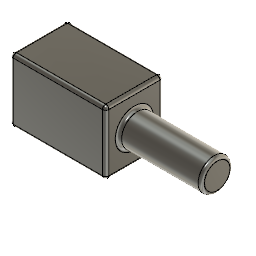
_Sign Holder (YIELD).780cf146-7897-4be0-9e8e-9a865215b20b (Autodesk Fusion 360 design; units mm, degrees)
Autodesk Fusion 360 part; units mm, degrees
sketch "Sketch1" plane through (0, 0, 0) normal (0, 0, 1) x (1, 0, 0)
  line L0 (0, 0) -> (-38.1, 0)
  line L1 (-38.1, 0) -> (-38.1, -38.1)
  line L2 (-38.1, -38.1) -> (0, -38.1)
  line L3 (0, -38.1) -> (0, 0)
  dimension "d1" = 38.1
  dimension "d2" = 38.1
  constraint horizontal L0
  constraint vertical L1
  constraint horizontal L2
  constraint vertical L3
  constraint coincident L0.start L3.end
  measures "d1" distance of L0.start L0.end
  measures "d2" distance of L0.start L2.end
extrude "Extrude1" add sketch "Sketch1" along normal blind 25.4
sketch "Sketch2" plane through (0, 0, 0) normal (1, 0, 0) x (0, 1, 0)
  line L0 (-38.1, 0) -> (0, 0)
  line L1 (0, 0) -> (0, 25.4)
  line L2 (0, 25.4) -> (-38.1, 25.4)
  line L3 (-38.1, 25.4) -> (-38.1, 0)
  line L4 (-38.1, 0) -> (-19.05, 0)
  line L5 (-19.05, 0) -> (-19.05, 12.7)
  circle A0 centre (-19.05, 12.7) radius 6.35
  dimension "d5" = 12.7
  constraint coincident L0.start L3.end
  constraint midpoint L0 L4.end
  constraint perpendicular L4 L5
  constraint coincident L5.end A0.centre
  measures "d5" diameter of A0
extrude "Extrude2" add sketch "Sketch2" along normal blind 12.7 contours A0
sketch "Sketch3" plane through (0, 0, 0) normal (0, 0, -1) x (1, 0, 0)
  line L0 (0, 0) -> (0, 38.1)
  line L1 (0, 38.1) -> (-38.1, 38.1)
  line L2 (-38.1, 38.1) -> (-38.1, 0)
  line L3 (-38.1, 0) -> (0, 0)
  line L4 (-38.1, 19.05) -> (-25.4, 19.05)
  line L5 (0, 19.05) -> (-12.7, 19.05)
  circle A0 centre (-12.7, 19.05) radius 3.175
  circle A1 centre (-25.4, 19.05) radius 3.175
  dimension "d9" = 12.7
  dimension "d10" = 12.7
  dimension "d11" = 6.35
  dimension "d12" = 6.35
  constraint midpoint L2 L4.start
  constraint perpendicular L2 L4
  constraint midpoint L0 L5.start
  constraint perpendicular L0 L5
  constraint coincident L5.end A0.centre
  constraint coincident L4.end A1.centre
  measures "d9" distance of L4.start L4.end
  measures "d10" distance of L5.start L5.end
  measures "d11" diameter of A0
  measures "d12" diameter of A1
extrude "Extrude3" add sketch "Sketch3" along normal blind 5.08 contours A1
extrude "Extrude4" add sketch "Sketch3" along normal blind 5.08 contours A0
extrude "Extrude5" cut 1 faces at (-12.7, 0, 8.4667) along direction (0, -1, 0) blind 7.62
extrude "Extrude6" cut 1 faces at (-25.4, -38.1, 8.4667) along direction (0, 1, 0) blind 7.62
extrude "Extrude7" cut 2 faces at (-13.6995, -18.8958, -5.08) (-24.8413, -17.3109, -5.08) along direction (0, 0, 1) blind 2.54
fillet "Fillet1" radius 1.27 12 faces at (-25.4, -30.48, 8.4667) (0, -18.8918, 2.1226) (-38.1, -15.24, 8.4667) (12.7, -19.3851, 13.862) (-12.7, -7.62, 8.4667) (-12.7, -22.86, 25.4) (4.2333, -12.7079, 13.0165) (-34.925, -19.05, 0) (-13.6995, -18.8958, -2.54) (-24.8413, -17.3109, -2.54) (-9.5408, -18.7339, -0.8467) (-22.2408, -19.3661, -1.6933)
delete_face "DeleteFace1" 1 faces at (11.8455, -21.9151, 7.1115)
extrude "Extrude8" add 1 faces at (12.7, -21.143, 15.8949) along direction (1, 0, 0) blind 20.32
fillet "Fillet2" radius 1.27 1 edges at (33.02, -24.9703, 10.4037)
equation "d6 = ( 1 / 2 ) * 1 in"
